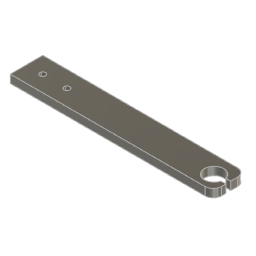
Light_cable_mount (Autodesk Fusion 360 design; units mm, degrees)
Autodesk Fusion 360 part; units mm, degrees
sketch "Sketch1" plane through (0, 0, 0) normal (0, 0, 1) x (1, 0, 0)
  line L0 (0, 0) -> (120, 0)
  line L1 (120, 20) -> (0, 20)
  line L2 (0, 20) -> (0, 0)
  line L3 (0, 10) -> (125, 9.2868) construction
  circle A0 centre (9.9998, 9.9429) radius 1.75
  circle A1 centre (25, 9.8574) radius 1.75
  arc A2 (125, 15) -> (120, 20) centre (120, 15) ccw
  arc A3 (120, 0) -> (125, 5) centre (120, 5) ccw
  line L4 (121.9893, 7.7868) -> (125, 7.7868)
  line L5 (125, 10.7868) -> (121.9893, 10.7868)
  line L6 (121.9893, 7.7868) -> (128.0107, 10.7868) construction
  line L7 (128.0107, 7.7868) -> (121.9893, 10.7868) construction
  line L8 (125, 5) -> (125, 7.7868)
  line L9 (125, 10.7868) -> (125, 15)
  arc A4 (122.0189, 10.772) -> (121.9893, 7.7868) centre (116.193, 9.337) ccw
  point P0 (125, 20)
  point P1 (125, 9.2868)
  dimension "d1" = 20
  dimension "d2" = 125
  dimension "d3" = 3.5
  dimension "d4" = 3.5
  dimension "d5" = 10
  dimension "d6" = 25
  dimension "d7" = 5
  dimension "d8" = 12
  dimension "d9" = 3
  constraint horizontal L0
  constraint vertical L8
  constraint horizontal L1
  constraint vertical L2
  constraint coincident L0.start L2.end
  constraint midpoint L2 L3.start
  constraint coincident L3 A0.centre
  constraint coincident L3 A1.centre
  constraint coincident P1 L8
  constraint coincident P0 L1
  constraint coincident P0 L8
  constraint tangent L1 A2
  constraint tangent A2 L8
  constraint tangent L0 A3
  constraint tangent A3 L8
  constraint equal A2 A3
  constraint coincident L3 A4.centre
  constraint horizontal L4
  constraint parallel L4 L5
  constraint coincident L6 P1
  constraint coincident L7 P1
  constraint coincident P1 L3.end
  constraint collinear L8 L9
  constraint coincident L7 A4.start
  measures "d1" distance of L0.start L1.end
  measures "d2" distance of P0 L1.end
  measures "d3" diameter of A0
  measures "d4" diameter of A1
  measures "d5" distance of L3.start A0.centre
  measures "d6" distance of L2 A1.centre
  measures "d7" radius of A2
  measures "d8" diameter of A4
  measures "d9" distance of L4 L5
extrude "Extrude1" add sketch "Sketch1" along normal blind 5
